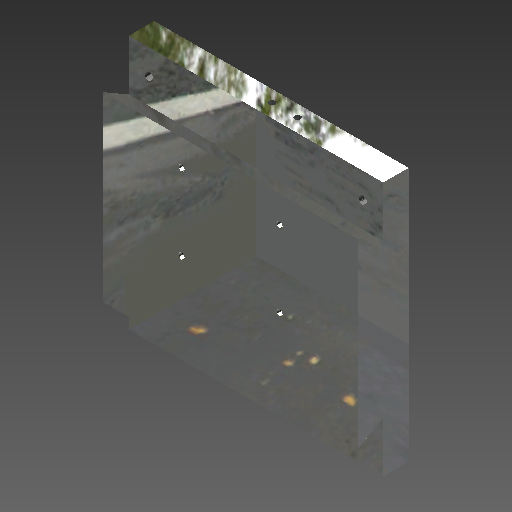
# Autodesk Inventor part: 3d_Welding_Tooling - Upper moving base
Saved by Autodesk Inventor 2018.3 (Build 223284000, 284)
## iProperties
Created: 2026-01-27
Part Number: 3d_Welding_Tooling - Upper moving base
Material: Aluminium 6061-T6
Document SubType Name: Modeling
Designer: aca6
Density: 2.7 g/cm^3
Appearance: N/A - Machined Aluminium
Manufacturer-1: {"Name": "Hanstar Technologies Co., Ltd", "PartNumber": "3d_Welding_Tooling - Upper moving base", "Link": ""}
Manufacturer-2: {"Name": "SHENZHEN JINYIHE PROTOTYPE TECHNOLOGIES CO., LTD", "PartNumber": "3d_Welding_Tooling - Upper moving base", "Link": ""}
Manufacturer-3: {"Name": "Shenzhen city Xavier Precision Co., Ltd.", "PartNumber": "3d_Welding_Tooling - Upper moving base", "Link": ""}
Manufacturer-4: {"Name": "", "PartNumber": "", "Link": ""}
Manufacturer-5: {"Name": "", "PartNumber": "", "Link": ""}
Provider-1: {"Name": "", "PartNumber": "", "Link": ""}
Provider-2: {"Name": "", "PartNumber": "", "Link": ""}
Provider-3: {"Name": "", "PartNumber": "", "Link": ""}
Provider-4: {"Name": "", "PartNumber": "", "Link": ""}
Provider-5: {"Name": "", "PartNumber": "", "Link": ""}
Author: aca6
Comments: DIN-ISO-2768-fH
Autodesk Inventor part; units mm, degrees
ref_plane "YZ Plane" through (0, 0, 0) normal (1, 0, 0) x (0, 1, 0)
ref_plane "XZ Plane" through (0, 0, 0) normal (0, 1, 0) x (-1, 0, 0)
ref_plane "XY Plane" through (0, 0, 0) normal (0, 0, 1) x (1, 0, 0)
sketch "Sketch1" plane through (0, 0, 0) normal (0, 0, 1) x (1, 0, 0)
  line L0 (-50, 50) -> (50, 50)
  line L1 (50, 50) -> (50, -50)
  line L2 (50, -50) -> (-50, -50)
  line L3 (-50, -50) -> (-50, 50)
  line L4 (0, 0) -> (0, 10.7535) construction
  line L5 (0, 0) -> (8.6992, 0) construction
  dimension "d0" = 100
  dimension "d1" = 100
  constraints: 12 end point, 3 horizontal, 2 parallel, 2 vertical, 1 perpendicular, 4 other
  measures "d0" distance of L0.start L0.end
  measures "d1" distance of L0.end L1.end
extrude "Extrusion1" add sketch "Sketch1" along normal blind 10
sketch "Sketch2" plane through (50, -50, 0) normal (1, 0, 0) x (0, 0, -1)
  line L0 (-10, 80) -> (-20, 85.7735)
  line L1 (-20, 85.7735) -> (-20, 14.2265)
  line L2 (-20, 14.2265) -> (-10, 20)
  line L3 (0, 0) -> (-10, 0) projected
  line L4 (0, 100) -> (-10, 100) projected
  line L5 (-10, 80) -> (-10, 20)
  line L6 (-10, 0) -> (-10, 100) projected
  point P0 (0, 50)
  dimension "d4" = 60
  dimension "d5" = 60
  dimension "d6" = 20
  dimension "d7" = 20
  dimension "d19" = 10
  constraints: 8 end point, 1 point on line, 1 vertical
  measures "d4" angle of L1 L0
  measures "d5" angle of L1 L2
  measures "d6" distance from line of L3 L2.end
  measures "d7" distance from line of L4 L0.start
  measures "d19" distance between parallel lines of L5 L1
extrude "Extrusion2" add sketch "Sketch2" against normal blind 100
sketch "Sketch3" plane through (0, 0, 0) normal (0, 0, -1) x (-1, 0, 0)
  circle A0 centre (19.25, -4.6808) radius 1.6 projected
  circle A1 centre (19.25, 25.3192) radius 1.6 projected
  circle A2 centre (-19.25, 25.3192) radius 1.6 projected
  circle A3 centre (-19.25, -4.6808) radius 1.6 projected
  point P0 (0, 0)
  constraints: 4 coincident
hole "Hole1" at (19.25, 25.3192, 0) at (19.25, -4.6808, 0) at (-19.25, 25.3192, 0) at (-19.25, -4.6808, 0) direction (0, 0, 1) diameter 2.459 end through all thread size "M3x0.5" class "6H" standard "ISO Metric profile"
sketch "Sketch4" plane through (0, 0, 0) normal (0, 0, -1) x (-1, 0, 0)
  line L0 (50, -50) -> (50, 50) projected
  line L1 (-50, -50) -> (50, -50) projected
  line L2 (50, 50) -> (-50, 50) projected
  line L3 (-50, 50) -> (-50, -50) projected
  point P0 (0, 0)
  point P1 (42, -40)
  point P2 (42, 40)
  point P3 (-42, 40)
  point P4 (-42, -40)
  dimension "d20" = 8
  dimension "d21" = 10
  dimension "d22" = 10
  dimension "d23" = 8
  constraints: 2 horizontal alignment, 2 vertical alignment
  measures "d20" distance from line of L0 point (42, -40)
  measures "d21" distance from line of L1 point (42, -40)
  measures "d22" distance from line of L2 point (42, 40)
  measures "d23" distance from line of L3 point (-42, -40)
hole "Hole2" at (-42, -40, 0) at (-42, 40, 0) at (42, 40, 0) at (42, -40, 0) direction (0, 0, 1) diameter 3.242 depth 11.8 tip angle 118 thread size "M4x0.7" class "6H" standard "ISO Metric profile"
chamfer "Chamfer1" distance 0.5 angle 45 4 edges at (-42, -41.621, 0) (-42, 38.379, 0) (42, 38.379, 0) (42, -41.621, 0)
sketch "Sketch5" plane through (-50, 50, 0) normal (0, 1, 0) x (1, 0, 0)
  circle A0 centre (51, -4.6715) radius 1.6 projected
  circle A1 centre (61, -4.6715) radius 1.6 projected
  point P0 (50, 0)
  constraints: 2 coincident
hole "Hole3" at (1, 50, 4.6715) at (11, 50, 4.6715) direction (0, -1, 0) diameter 2.459 depth 13 tip angle 118 thread size "M3x0.5" class "6H" standard "ISO Metric profile"
body "Solid1"
